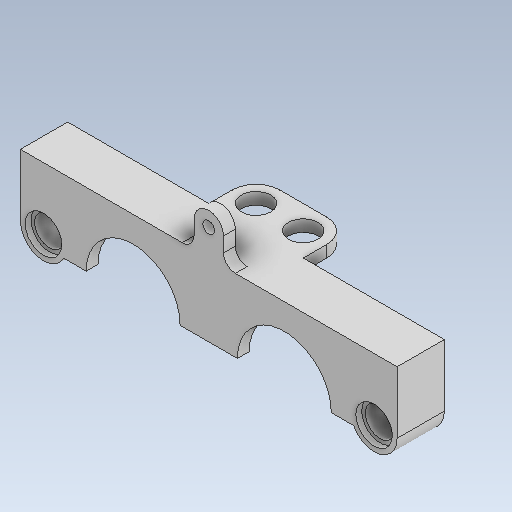
# Autodesk Inventor part: apoio ultrassonico
Saved by Autodesk Inventor 2020 (Build 240168000, 168)
## iProperties
Created: 2020-04-22
Part Number: apoio ultrassonico
Material: Genérico
Document SubType Name: Modeling
Designer: gi-se
Density: 1 g/cm^3
Appearance: Padrão
Author: gi-se
Autodesk Inventor part; units mm, degrees
ref_plane "YZ Plane" through (0, 0, 0) normal (1, 0, 0) x (0, 1, 0)
ref_plane "XZ Plane" through (0, 0, 0) normal (0, 1, 0) x (-1, 0, 0)
ref_plane "XY Plane" through (0, 0, 0) normal (0, 0, 1) x (1, 0, 0)
sketch "Esboço1" plane through (0, 0, 0) normal (0, 0, 1) x (1, 0, 0)
  circle A0 centre (8.001, 0) radius 2.4 projected
  circle A1 centre (8.001, 0) radius 2.4
  circle A2 centre (64.001, 0) radius 2.4 projected
  circle A3 centre (64.001, 0) radius 2.4
  line L0 (58.601, 8.5) -> (13.401, 8.5) projected
  line L1 (58.601, -12.1) -> (58.601, 8.5) projected
  line L2 (13.401, 8.5) -> (13.401, -12.1) projected
  line L3 (67.806, 3.9) -> (60.196, 3.9) projected
  arc A4 (60.101, 0) -> (67.901, 0) centre (64.001, 0) ccw
  line L4 (60.101, 0) -> (60.101, 8.5)
  line L5 (60.101, 8.5) -> (11.901, 8.5)
  arc A5 (4.101, 0) -> (11.901, 0) centre (8.001, 0) ccw
  line L6 (11.901, 0) -> (11.901, 8.5)
  line L7 (4.101, 0) -> (4.101, 8.5)
  line L8 (4.101, 8.5) -> (4.101, 10.5)
  line L9 (67.901, 0) -> (67.901, 10.2879)
  line L10 (67.901, 10.5) -> (4.101, 10.5)
  line L11 (67.901, 10.1485) -> (67.901, 10.5)
  point P0 (0, 0)
  dimension "d0" = 7.8
  dimension "d1" = 2
  constraints: 16 end point, 6 coincident, 4 centre point, 4 point on circle, 4 tangent, 3 vertical, 2 concentric, 2 perpendicular, 1 horizontal, 1 parallel, 1 point on line
  measures "d0" diameter of A5
  measures "d1" distance of L7.end L8.end
extrude "Extrusão1" add sketch "Esboço1" along normal blind 8
sketch "Esboço3" plane through (0, 0, 8) normal (0, 0, 1) x (1, 0, 0)
  circle A0 centre (23.201, -1.8) radius 7.95 projected
  circle A1 centre (48.801, -1.8) radius 7.95 projected
  arc A2 (60.101, 0) -> (67.901, 0) centre (64.001, 0) ccw projected
  line L0 (11, -1.8) -> (11, 9)
  line L1 (11, 9) -> (60.5412, 9)
  line L2 (60.5412, 9) -> (60.5412, -1.8)
  line L3 (15.251, -1.8) -> (11, -1.8)
  line L4 (60.5412, -1.8) -> (56.751, -1.8)
  line L5 (40.851, -1.8) -> (31.151, -1.8)
  point P0 (0, 0)
  constraints: 12 end point, 5 point on circle, 4 parallel, 3 horizontal, 3 perpendicular
extrude "Extrusão2" add sketch "Esboço3" against normal blind 2 contours A0 L3 L0 L1 L2 L4 A1 L5
sketch "Esboço4" plane through (0, 0, 8) normal (0, 0, 1) x (1, 0, 0)
  circle A0 centre (8, 0) radius 3.1
  circle A1 centre (64.001, 0) radius 2.4 projected
  circle A2 centre (64, 0) radius 3.1
  circle A3 centre (8.001, 0) radius 2.4 projected
  point P0 (0, 0)
  dimension "d6" = 6.2
  dimension "d7" = 6.2
  constraints: 2 centre point
  measures "d6" diameter of A0
  measures "d7" diameter of A2
extrude "Extrusão3" cut sketch "Esboço4" against normal blind 1
sketch "Esboço5" plane through (0, 0, 0) normal (0, 0, -1) x (-1, 0, 0)
  circle A0 centre (-8, 0) radius 3.1
  circle A1 centre (-8.001, 0) radius 2.4 projected
  circle A2 centre (-64.001, 0) radius 2.4 projected
  circle A3 centre (-64.001, 0) radius 3.1 projected
  point P0 (0, 0)
  dimension "d10" = 6.2
  constraints: 1 centre point
  measures "d10" diameter of A0
extrude "Extrusão4" cut sketch "Esboço5" against normal blind 1
sketch "Esboço6" plane through (0, 0, 8) normal (0, 0, 1) x (1, 0, 0)
  line L0 (33.501, 12.5) -> (33.501, 15)
  line L1 (38.501, 15) -> (38.501, 12.5)
  line L2 (4.101, 10.5) -> (4.101, 0) projected
  line L3 (-3.999, -3.9) -> (-3.999, 3.9) projected
  circle A0 centre (36.001, 15) radius 1
  circle A1 centre (36.001, 15) radius 2.5
  arc A2 (31.501, 10.5) -> (33.501, 12.5) centre (31.501, 12.5) ccw
  arc A3 (38.501, 12.5) -> (40.501, 10.5) centre (40.501, 12.5) ccw
  line L4 (40.501, 10.5) -> (31.501, 10.5)
  line L5 (67.901, 10.5) -> (4.101, 10.5) projected
  point P0 (0, 0)
  dimension "d19" = 29.4
  dimension "d20" = 2
  dimension "d22" = 2
  dimension "d23" = 2
  constraints: 6 end point, 6 point on circle, 4 centre point, 4 tangent, 1 coincident, 1 collinear
  measures "d19" distance between parallel lines of L2 L0
  measures "d20" diameter of A0
  measures "d22" radius of A2
  measures "d23" radius of A3
extrude "Extrusão5" add sketch "Esboço6" against normal blind 2
sketch "Esboço8" plane through (0, 0, 0) normal (0, 0, -1) x (-1, 0, 0)
  line L0 (-28.001, 3.9) -> (-28.001, 3.6) projected
  line L1 (-11.901, 8.5) -> (-60.101, 8.5) projected
  line L2 (-67.901, 10.5) -> (-4.101, 10.5) projected
  line L3 (-28.001, 8.5) -> (-44.001, 8.5)
  line L4 (-44.001, 8.5) -> (-44.001, 10.5)
  line L5 (-44.001, 10.5) -> (-28.001, 10.5)
  line L6 (-28.001, 10.5) -> (-28.001, 8.5)
  point P0 (0, 0)
  dimension "d24" = 16
  constraints: 8 end point, 2 parallel, 2 point on line, 1 horizontal, 1 perpendicular
  measures "d24" distance of L4.end L5.end
extrude "Extrusão6" add sketch "Esboço8" along normal blind 8
sketch "Esboço9" plane through (11.901, 8.5, 6) normal (0, -1, 0) x (1, 0, 0)
  circle A0 centre (28.1, -10) radius 2.4 projected
  circle A1 centre (20.1, -10) radius 2.4 projected
  arc A2 (16.1, -10) -> (20.1, -14) centre (20.1, -10) ccw
  line L0 (32.1, -14) -> (16.1, -14) projected
  arc A3 (28.1, -14) -> (32.1, -10) centre (28.1, -10) ccw
  line L1 (32.1, -6) -> (32.1, -14) projected
  line L2 (16.1, -10) -> (16.1, -14)
  line L3 (32.1, -14) -> (32.1, -10)
  line L4 (16.1, -14) -> (20.1, -14)
  line L5 (28.1, -14) -> (32.1, -14)
  point P0 (-11.901, -6)
  point P1 (28.1, -14)
  constraints: 8 end point, 4 point on circle, 2 centre point, 2 coincident, 2 tangent, 1 midpoint, 1 parallel
extrude "Extrusão7" cut sketch "Esboço9" against normal blind 6.75
sketch "Esboço10" plane through (64.001, 0, 1) normal (0, 0, -1) x (-1, 0, 0)
  circle A0 centre (0, 0) radius 2.4 projected
  circle A1 centre (56, 0) radius 2.4 projected
  circle A2 centre (0, 0) radius 2.5
  circle A3 centre (56, 0) radius 2.5
  point P0 (64.001, 0)
  dimension "d29" = 5
  dimension "d30" = 5
  constraints: 2 centre point, 2 coincident
  measures "d29" diameter of A2
  measures "d30" diameter of A3
extrude "Extrusão8" cut sketch "Esboço10" against normal blind 15.25
sketch "Esboço11" plane through (4.101, 10.5, 8) normal (0, 1, 0) x (1, 0, 0)
  circle A0 centre (27.9, 12) radius 2.4 projected
  circle A1 centre (35.9, 12) radius 2.4 projected
  circle A2 centre (27.9, 12) radius 2.5
  circle A3 centre (35.9, 12) radius 2.5
  point P0 (-4.101, 8)
  dimension "d33" = 5
  dimension "d34" = 5
  constraints: 2 centre point, 2 coincident
  measures "d33" diameter of A2
  measures "d34" diameter of A3
extrude "Extrusão9" cut sketch "Esboço11" against normal blind 10
